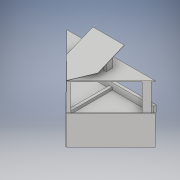
# Autodesk Inventor part: Barn and Rad
Saved by Autodesk Inventor 2017 (Build 210142000, 142)
## iProperties
Created: 2017-04-14
Part Number: Barn and Rad
Material: Generic
Document SubType Name: Modeling
Designer: Alex Tacescu
Density: 1 g/cm^3
Appearance: Default
Author: Alex Tacescu
Autodesk Inventor part; units mm, degrees
ref_plane "YZ Plane" through (0, 0, 0) normal (1, 0, 0) x (0, 1, 0)
ref_plane "XZ Plane" through (0, 0, 0) normal (0, 1, 0) x (-1, 0, 0)
ref_plane "XY Plane" through (0, 0, 0) normal (0, 0, 1) x (1, 0, 0)
sketch "Sketch1" plane through (0, 0, 0) normal (0, 1, 0) x (-1, 0, 0)
  line L0 (0, -122.3426) -> (0, 734.0556) projected
  line L1 (-853.44, 0) -> (853.44, 0) projected
  line L2 (609.6, 0) -> (-609.6, 0)
  line L3 (-609.6, 0) -> (0, 611.713)
  line L4 (0, 611.713) -> (609.6, 0)
  point P0 (0, 0)
  dimension "d0" = 1219.2
  dimension "d1" = 609.6
  dimension "d2" = 863.6
  constraints: 6 end point, 3 point on line
  measures "d0" distance of L2.start L2.end
  measures "d1" distance from line of L0 L2.start
  measures "d2" distance of L3.end L2.start
extrude "Extrusion1" add sketch "Sketch1" along normal blind 381
sketch "Sketch4" plane through (0, 0, 611.713) normal (-0.7083291, 0, 0.7058824) x (0.7058824, 0, 0.7083291)
  line L0 (-863.6, 0) -> (0, 0) projected
  line L1 (0, 0) -> (0, 381) projected
  line L2 (-863.6, 381) -> (0, 381) projected
  line L3 (-863.6, 0) -> (-863.6, 381) projected
  line L4 (-863.6, 381) -> (0, 381)
  line L5 (0, 381) -> (0, 406.4)
  line L6 (0, 406.4) -> (-863.6, 406.4)
  line L7 (-863.6, 406.4) -> (-863.6, 381)
  line L8 (-863.6, 0) -> (-863.6, 381) projected
  point P0 (-433.2941, 0)
  dimension "d7" = 25.4
  constraints: 8 end point, 3 collinear, 2 parallel, 1 horizontal, 1 perpendicular
  measures "d7" distance of L6.end L4.start
extrude "Extrusion3" add sketch "Sketch4" along normal blind 6.35
mirror "Mirror2" about plane through (0, 0, 0) normal (1, 0, 0) of "Extrusion3"
sketch "Sketch5" plane through (0, 381, 0) normal (0, 1, 0) x (1, 0, 0)
  line L0 (0, -611.713) -> (609.6, 0) projected
  line L1 (609.6, 0) -> (-609.6, 0) projected
  line L2 (-609.6, 0) -> (0, -611.713) projected
  line L3 (-584.2, 0) -> (584.2, 0)
  line L4 (584.2, 0) -> (584.2, 38.1)
  line L5 (584.2, 38.1) -> (-584.2, 38.1)
  line L6 (-584.2, 38.1) -> (-584.2, 0)
  point P0 (0, 0)
  dimension "d10" = 1168.4
  dimension "d11" = 584.2
  dimension "d12" = 38.1
  constraints: 8 end point, 2 parallel, 1 horizontal, 1 perpendicular, 1 point on line
  measures "d10" distance of L4.end L5.end
  measures "d11" distance from line of point (0, 0) L6
  measures "d12" distance of L5.end L3.start
extrude "Extrusion4" add sketch "Sketch5" along normal blind 88.9 contours L1 L6 L5 L4
sketch "Sketch6" plane through (0, 381, 0) normal (0, 1, 0) x (1, 0, 0)
  line L0 (0, -611.713) -> (609.6, 0) projected
  line L1 (609.6, 0) -> (584.2, 0) projected
  line L2 (584.2, 0) -> (-584.2, 0) projected
  line L3 (-584.2, 0) -> (-609.6, 0) projected
  line L4 (-609.6, 0) -> (0, -611.713) projected
  line L5 (0, 168.9591) -> (0, -747.0544) projected
  line L6 (19.05, -558.8) -> (-19.05, -558.8)
  line L7 (-19.05, -558.8) -> (-19.05, 0)
  line L8 (-19.05, 0) -> (19.05, 0)
  line L9 (19.05, 0) -> (19.05, -558.8)
  line L10 (19.05, -558.8) -> (-19.05, 0) construction
  line L11 (-19.05, -558.8) -> (19.05, 0) construction
  point P0 (0, 0)
  point P1 (0, -279.4)
  dimension "d15" = 38.1
  dimension "d16" = 558.8
  constraints: 12 end point, 2 midpoint, 2 parallel, 2 point on line, 1 horizontal, 1 perpendicular
  measures "d15" distance of L6.start L6.end
  measures "d16" distance of L8.end L6.start
extrude "Extrusion5" add sketch "Sketch6" along normal blind 38.1 contours L6 L7 L2 L5 | L5 L2 L9 L6
sketch "Sketch7" plane through (0, 381, 0) normal (0, 1, 0) x (1, 0, 0)
  line L0 (609.6, 0) -> (-609.6, 0) projected
  line L1 (609.6, 0) -> (614.0979, -4.4824) projected
  line L2 (614.0979, -4.4824) -> (4.4979, -616.1954) projected
  line L3 (0, -611.713) -> (4.4979, -616.1954) projected
  line L4 (0, -611.713) -> (-4.4979, -616.1954) projected
  line L5 (-614.0979, -4.4824) -> (-4.4979, -616.1954) projected
  line L6 (-609.6, 0) -> (-614.0979, -4.4824) projected
  line L7 (0, 168.9591) -> (0, -747.0544) projected
  line L8 (0, -611.713) -> (26.9408, -584.7722)
  line L9 (26.9408, -584.7722) -> (0, -557.8315)
  line L10 (0, -557.8315) -> (-26.9408, -584.7722)
  line L11 (-26.9408, -584.7722) -> (0, -611.713)
  line L12 (555.8114, 0) -> (582.7988, -26.8941)
  line L13 (582.7988, -26.8941) -> (520.0458, -89.8646)
  line L14 (520.0458, -89.8646) -> (493.0585, -62.9705)
  line L15 (493.0585, -62.9705) -> (555.8114, 0)
  line L16 (-555.8114, 0) -> (-582.7988, -26.8941)
  line L17 (-582.7988, -26.8941) -> (-520.0458, -89.8646)
  line L18 (-520.0458, -89.8646) -> (-493.0585, -62.9705)
  line L19 (-493.0585, -62.9705) -> (-555.8114, 0)
  point P0 (0, 0)
  dimension "d19" = 38.1
  dimension "d20" = 88.9
  dimension "d21" = 38.1
  dimension "d22" = 6.35
  constraints: 24 end point, 5 parallel, 4 symmetric about line, 3 perpendicular, 2 point on line
  measures "d19" distance of L9.end L10.end
  measures "d20" distance of L14.end L12.start
  measures "d21" distance of L13.end L14.end
  measures "d22" distance between parallel lines of L2 L13
extrude "Extrusion6" add sketch "Sketch7" along normal blind 393.7 contours L12 L13 L14 L15 | L19 L18 L17 L16 | L9 L8 L7 | L7 L11 L10
sketch "Sketch8" plane through (0, 774.7, 0) normal (0, 1, 0) x (1, 0, 0)
  line L0 (-520.0458, -89.8646) -> (-493.0585, -62.9705) projected
  line L1 (-493.0585, -62.9705) -> (-555.8114, 0) projected
  line L2 (-555.8114, 0) -> (-582.7988, -26.8941) projected
  line L3 (-582.7988, -26.8941) -> (-520.0458, -89.8646) projected
  line L4 (555.8114, 0) -> (493.0585, -62.9705) projected
  line L5 (493.0585, -62.9705) -> (520.0458, -89.8646) projected
  line L6 (520.0458, -89.8646) -> (582.7988, -26.8941) projected
  line L7 (582.7988, -26.8941) -> (555.8114, 0) projected
  line L8 (0, -611.713) -> (26.9408, -584.7722) projected
  line L9 (26.9408, -584.7722) -> (0, -557.8315) projected
  line L10 (0, -557.8315) -> (-26.9408, -584.7722) projected
  line L11 (-26.9408, -584.7722) -> (0, -611.713) projected
  line L12 (-609.6, 0) -> (609.6, 0)
  line L13 (609.6, 0) -> (0, -611.713)
  line L14 (0, -611.713) -> (-609.6, 0)
  line L15 (0, 168.9591) -> (0, -747.0544) projected
  point P0 (0, 0)
  dimension "d25" = 863.6
  dimension "d26" = 1219.2
  constraints: 6 end point, 1 equal length, 1 horizontal
  measures "d25" distance of L8.start L12.start
  measures "d26" distance of L12.start L12.end
extrude "Extrusion7" add sketch "Sketch8" along normal blind 12.7 contours L3 L2 L1 L0 | L0 L1 L12 L15 L10 L14 | L14 L12 L2 | L10 L15 L14 | L15 L12 L4 L5 L13 L9 | L9 L13 L15 | L7 L6 L5 L4 | L12 L13 L7
sketch "Sketch9" plane through (0, 787.4, 0) normal (0, 1, 0) x (1, 0, 0)
  line L0 (0, -611.713) -> (609.6, 0) projected
  line L1 (609.6, 0) -> (-609.6, 0) projected
  line L2 (-609.6, 0) -> (0, -611.713) projected
  line L3 (0, 168.9591) -> (0, -747.0544) projected
  line L4 (127, -139.7) -> (165.1, -139.7)
  line L5 (165.1, -139.7) -> (165.1, -228.6)
  line L6 (165.1, -228.6) -> (127, -228.6)
  line L7 (127, -228.6) -> (127, -139.7)
  point P0 (0, 0)
  dimension "d29" = 139.7
  dimension "d30" = 38.1
  dimension "d31" = 88.9
  dimension "d43" = 165.1
  constraints: 8 end point, 2 parallel, 1 horizontal, 1 perpendicular
  measures "d29" distance between parallel lines of L1 L4
  measures "d30" distance of L4.start L4.end
  measures "d31" distance of L4.end L5.end
  measures "d43" distance between parallel lines of L5 L3
extrude "Extrusion8" add sketch "Sketch9" along normal blind 158.75 contours L4 L5 L6 L7
sketch "Sketch10" plane through (165.1, 787.4, 228.6) normal (1, 0, 0) x (0, 0, -1)
  line L0 (88.9, 0) -> (0, 0) projected
  line L1 (88.9, 0) -> (88.9, 158.75) projected
  line L2 (0, 158.75) -> (88.9, 158.75) projected
  line L3 (0, 0) -> (0, 158.75) projected
  line L4 (0, 158.75) -> (88.9, 195.5736)
  line L5 (88.9, 195.5736) -> (88.9, 158.75)
  point P0 (228.6, -787.4)
  dimension "d35" = 112.5
  constraints: 4 end point, 1 collinear
  measures "d35" angle of L3 L4
extrude "Extrusion9" add sketch "Sketch10" against normal up to surface (38.1 mm away) contours L2 L4 L5
mirror "Mirror3" about plane through (0, 0, 0) normal (1, 0, 0) of "Extrusion8", "Extrusion9"
sketch "Sketch11" plane through (-165.1, 982.9736, 139.7) normal (0, 0.9238795, 0.3826834) x (1, 0, 0)
  line L0 (38.1, 0) -> (38.1, -96.2247) projected
  line L1 (0, 0) -> (38.1, 0) projected
  line L2 (0, 0) -> (0, -96.2247) projected
  line L3 (38.1, -96.2247) -> (0, -96.2247) projected
  line L4 (292.1, 0) -> (292.1, -96.2247) projected
  line L5 (292.1, -96.2247) -> (330.2, -96.2247) projected
  line L6 (330.2, 0) -> (330.2, -96.2247) projected
  line L7 (330.2, 0) -> (292.1, 0) projected
  line L8 (0, -156.9757) -> (0, -74.8428) projected
  line L9 (0, -74.8428) -> (38.1, -74.8428) projected
  line L10 (38.1, -74.8428) -> (38.1, -156.9757) projected
  line L11 (38.1, -156.9757) -> (0, -156.9757) projected
  line L12 (330.2, -74.8428) -> (330.2, -156.9757) projected
  line L13 (330.2, -156.9757) -> (292.1, -156.9757) projected
  line L14 (292.1, -156.9757) -> (292.1, -74.8428) projected
  line L15 (292.1, -74.8428) -> (330.2, -74.8428) projected
  line L16 (165.1, -510.9259) -> (774.7, 54.2232) projected
  line L17 (774.7, 54.2232) -> (-444.5, 54.2232) projected
  line L18 (-444.5, 54.2232) -> (165.1, -510.9259) projected
  line L19 (-50.8, 117.7241) -> (-50.8, -275.9759)
  line L20 (-50.8, -275.9759) -> (165.1, -510.9259)
  line L21 (165.1, 381.0857) -> (165.1, -1015.9716) projected
  line L22 (-50.8, 117.7241) -> (165.1, 117.7241)
  line L23 (381, 117.7241) -> (381, -275.9759)
  line L24 (381, -275.9759) -> (165.1, -510.9259)
  line L25 (381, 117.7241) -> (165.1, 117.7241)
  point P0 (165.1, -247.1017)
  dimension "d38" = 393.7
  dimension "d39" = 234.95
  dimension "d40" = 215.9
  constraints: 12 end point, 2 perpendicular, 2 symmetric about line, 1 point on line
  measures "d38" distance of L19.start L19.end
  measures "d39" vertical distance of L16.start L19.end
  measures "d40" distance of L19.start L22.end
extrude "Extrusion10" add sketch "Sketch11" along normal blind 6.35 contours L0 L9 L2 L1 | L0 L3 L2 L9 | L10 L11 L8 L3 | L7 L6 L15 L4 | L15 L6 L5 L4 | L5 L12 L13 L14 | L20 L19 L17 L21 | L21 L17 L23 L24 | L21 L25 L23 L17 | L17 L19 L22 L21
equation "\"d1\" = 0.5 * d0"
equation "\"d11\" = 0.5 * d10"
body "Solid1"
